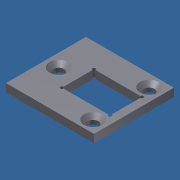
# Autodesk Inventor part: ASSOALHO(8)
Saved by Autodesk Inventor 2012 SP1 (Build 160190100, 190)
## iProperties
Created: 2012-07-23
Part Number: ASSOALHO(8)
Material: Carbon Steel
Document SubType Name: Modeling
Designer: bruno.silveira
Mass: 108.213 g
Surface Area: 65.5 cm^2
Volume: 13.75 cm^3
Density: 7.87 g/cm^3
Author: bruno.silveira
Autodesk Inventor part; units mm, degrees
ref_plane "YZ Plane" through (0, 0, 0) normal (1, 0, 0) x (0, 1, 0)
ref_plane "XZ Plane" through (0, 0, 0) normal (0, 1, 0) x (-1, 0, 0)
ref_plane "XY Plane" through (0, 0, 0) normal (0, 0, 1) x (1, 0, 0)
sketch "Sketch1" plane through (0, 0, 0) normal (0, 0, 1) x (1, 0, 0)
  line L0 (0, 0) -> (55, 0)
  line L1 (55, 0) -> (55, 50)
  line L2 (55, 50) -> (0, 50)
  line L3 (0, 50) -> (0, 0)
  dimension "d0" = 55
  dimension "d1" = 50
  constraints: 8 end point, 2 parallel, 1 horizontal, 1 perpendicular
  measures "d0" distance of L1.end L2.end
  measures "d1" distance of L2.end L0.start
extrude "Extrusion1" add sketch "Sketch1" along normal blind 5
sketch "Sketch2" plane through (0, 0, 5) normal (0, 0, 1) x (1, 0, 0)
  line L0 (55, 0) -> (0, 0) projected
  line L1 (55, 50) -> (55, 0) projected
  line L2 (20, 15) -> (50, 15)
  line L3 (50, 15) -> (50, 35)
  line L4 (50, 35) -> (20, 35)
  line L5 (20, 35) -> (20, 15)
  dimension "d4" = 30
  dimension "d5" = 20
  dimension "d6" = 5
  dimension "d7" = 15
  constraints: 8 end point, 2 parallel, 1 horizontal, 1 perpendicular
  measures "d4" distance of L2.start L2.end
  measures "d5" distance of L2.end L3.end
  measures "d6" distance between parallel lines of L1 L3
  measures "d7" distance between parallel lines of L0 L2
extrude "Extrusion2" cut sketch "Sketch2" against normal blind 5
sketch "Sketch3" plane through (0, 0, 5) normal (0, 0, 1) x (1, 0, 0)
  circle A0 centre (20, 35) radius 1
  circle A1 centre (20, 15) radius 1
  circle A2 centre (50, 15) radius 1
  circle A3 centre (50, 35) radius 1
  point P0 (50, 35)
  point P1 (20, 15)
  dimension "d10" = 2
  dimension "d11" = 2
  dimension "d12" = 2
  dimension "d13" = 2
  constraints: 4 centre point, 1 coincident
  measures "d10" diameter of A0
  measures "d11" diameter of A1
  measures "d12" diameter of A2
  measures "d13" diameter of A3
hole "Hole1" at (20, 35, 5) at (20, 15, 5) at (50, 15, 5) at (50, 35, 5) direction (0, 0, -1) diameter 2 depth 5 tip angle 118
sketch "Sketch4" plane through (0, 0, 5) normal (0, 0, 1) x (1, 0, 0)
  line L0 (0, 0) -> (0, 50) projected
  line L1 (55, 0) -> (0, 0) projected
  line L2 (55, 50) -> (55, 0) projected
  line L3 (0, 50) -> (55, 50) projected
  point P0 (8, 25)
  point P1 (47, 42.5)
  point P2 (47, 7.5)
  dimension "d21" = 35
  dimension "d22" = 7.5
  dimension "d23" = 8
  dimension "d24" = 8
  dimension "d25" = 8
  dimension "d26" = 25
  measures "d21" distance of point (47, 7.5) point (47, 42.5)
  measures "d22" distance from line of L1 point (47, 7.5)
  measures "d23" distance from line of L2 point (47, 42.5)
  measures "d24" distance from line of L2 point (47, 7.5)
  measures "d25" distance from line of L0 point (8, 25)
  measures "d26" distance from line of L3 point (8, 25)
hole "Hole2" at (8, 25, 5) at (47, 42.5, 5) at (47, 7.5, 5) direction (0, 0, -1) diameter 6.5 depth 5 tip angle 118 countersink diameter 11.5 countersink angle 90
body "Solid1"
